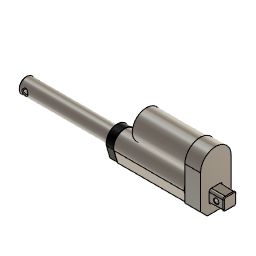
сборка v7 (Autodesk Fusion 360 archive; units mm, degrees)
design "actuators 10"
Autodesk Fusion 360 part; units mm, degrees
note: some values were not read from the file. Set by a fixed rule: which face or edge a step refers to.
sketch "Sketch1" plane through (0, 0, 0) normal (0, 0, 1) x (1, 0, 0)
  line L0 (8.5, 8.5) -> (-8.5, 8.5)
  line L1 (-8.5, 8.5) -> (-8.5, -8.5)
  line L2 (-8.5, -8.5) -> (8.5, -8.5)
  line L3 (8.5, -8.5) -> (8.5, 8.5)
  line L4 (8.5, 8.5) -> (-8.5, -8.5) construction
  line L5 (-8.5, 8.5) -> (8.5, -8.5) construction
  dimension "d1" = 17
  dimension "d2" = 17
  constraint horizontal L0
  constraint perpendicular L0 L1
  constraint parallel L0 L2
  constraint parallel L1 L3
  constraint coincident L4 origin
  constraint coincident L5 origin
  measures "d1" distance of L1.end L2.end
  measures "d2" distance of L0.end L1.end
ref_plane "WorkPlane1" through (0, 0, 19) normal (0, 0, 1) x (1, 0, 0)
sketch "Sketch2" plane through (0, 0, 19) normal (0, 0, 1) x (1, 0, 0)
  line L0 (9, 9) -> (-9, 9)
  line L1 (-9, 9) -> (-9, -9)
  line L2 (-9, -9) -> (9, -9)
  line L3 (9, -9) -> (9, 9)
  line L4 (9, 9) -> (-9, -9) construction
  line L5 (-9, 9) -> (9, -9) construction
  dimension "d4" = 18
  dimension "d5" = 18
  constraint horizontal L0
  constraint perpendicular L0 L1
  constraint parallel L0 L2
  constraint parallel L1 L3
  constraint coincident L4 origin
  constraint coincident L5 origin
  measures "d4" distance of L1.end L2.end
  measures "d5" distance of L0.end L1.end
loft "Loft1" add profiles "Sketch1", "Sketch2" section 1 section 2 makes body 1
fillet "Fillet1" radius 3 4 edges at (8.75, -8.75, 9.5) (-8.75, -8.75, 9.5) (-8.75, 8.75, 9.5) (8.75, 8.75, 9.5) on bodies 1
fillet "Fillet2" radius 1 1 faces at (-1.8337, -2.8333, 0) on bodies 1
sketch "Sketch3" plane through (0, 8.4941, -0.2235) normal (0, 0.999654, -0.026307) x (-1, 0, 0)
  line L0 (-5.5267, 1.1976) -> (5.5267, 1.1976)
  line L1 (5.5267, 1.1976) -> (6.001, 19.2302)
  line L2 (6.001, 19.2302) -> (-6.001, 19.2302)
  line L3 (-6.001, 19.2302) -> (-5.5267, 1.1976)
  line L4 (0, 0) -> (0, 6.5)
  line L5 (0, 6.5) -> (0.0789, 9.499)
  circle A0 centre (0.0789, 9.499) radius 3
  dimension "d10" = 6.5
  dimension "d11" = 3
  constraint coincident L4.start origin
  constraint perpendicular L0 L4
  constraint parallel L1 L5
  constraint coincident L5.end A0.centre
  constraint coincident L4.end A0
  measures "d10" distance of L4.start L4.end
  measures "d11" distance of L4.end L5.end
extrude "Extrude1" cut sketch "Sketch3" against normal blind 32 contours A0 bodies 1
fillet "Fillet3" radius 0.5 2 edges at (-0.0789, -8.8352, 12.7358) (2.7181, 8.7725, 10.3566) on bodies 1
sketch "Sketch4" plane through (0, 0, 19) normal (0, 0, 1) x (-1, 0, 0)
  ellipse E0 centre (-5.999, -5.999) end of major axis (-8.1218, -8.1218) minor radius 3 (-9, -6.001) -> (-6.001, -9) ccw
  line L0 (-6.001, -9) -> (6.001, -9)
  ellipse E1 centre (5.999, -5.999) end of major axis (8.1218, -8.1218) minor radius 3 (6.001, -9) -> (9, -6.001) ccw
  line L1 (9, -6.001) -> (9, 6.001)
  ellipse E2 centre (5.999, 5.999) end of major axis (8.1218, 8.1218) minor radius 3 (9, 6.001) -> (6.001, 9) ccw
  line L2 (6.001, 9) -> (-6.001, 9)
  ellipse E3 centre (-5.999, 5.999) end of major axis (-8.1218, 8.1218) minor radius 3 (-6.001, 9) -> (-9, 6.001) ccw
  line L3 (-9, 6.001) -> (-9, -6.001)
  line L4 (9, 0) -> (20.5, 0)
  line L5 (20.5, 0) -> (20.5, -11.5)
  line L6 (0, 0) -> (-39.2189, 0) construction
  line L7 (0, 0) -> (0, -20.5) construction
  line L8 (0, -20.5) -> (-34, -20.5)
  line L9 (20.5, -11.5) -> (11.5, -20.5)
  line L10 (20.5, -11.5) -> (33.2279, -11.5) construction
  line L11 (0, -20.5) -> (11.5, -20.5)
  line L12 (-54.5, 0) -> (-54.5, 0)
  arc A0 (-54.5, 0) -> (-34, -20.5) centre (-34, 0) ccw
  line L13 (20.5, 11.5) -> (11.5, 20.5)
  line L14 (20.5, 0) -> (20.5, 11.5)
  line L15 (0, 20.5) -> (11.5, 20.5)
  line L16 (0, 20.5) -> (-34, 20.5)
  arc A1 (-34, 20.5) -> (-54.5, 0) centre (-34, 0) ccw
  dimension "d16" = 11.5
  dimension "d17" = 11.5
  dimension "d19" = 20.5
  dimension "d23" = 135
  dimension "d25" = 20.5
  constraint midpoint L1 L4.start
  constraint perpendicular L1 L4
  constraint perpendicular L4 L5
  constraint coincident L6.start L7.start
  constraint horizontal L6
  constraint perpendicular L6 L7
  constraint perpendicular L7 L8
  constraint horizontal L10
  constraint tangent L8 A0
  constraint symmetric L4.end L6 L5.start
  constraint symmetric L5.end L6 L13.start
  constraint symmetric L6 L7.end L15.start
  constraint symmetric L6 L9.end L13.end
  constraint symmetric L6 L8.end L16.end
  constraint symmetric L6 L12.start L12.end
  constraint symmetric L6 A0 A1
  measures "d16" distance of L4.start L4.end
  measures "d17" distance of L4.end L5.end
  measures "d19" distance of L6.start L7.end
  measures "d23" angle of L9 L10
  measures "d25" radius of A0
extrude "Extrude2" add sketch "Sketch4" along normal blind 21 contours E0 L0 E1 L1 E2 L2 E3 L3 | L5 L8 L9 L11 A0 L13 L14 L15 L16 A1 bodies 1
sketch "Sketch5" plane through (0, 0, 40) normal (0, 0, 1) x (-1, 0, 0)
  line L0 (11.5, 20.5) -> (-34, 20.5)
  arc A0 (-34, 20.5) -> (-34, -20.5) centre (-34, 0) ccw
  line L1 (-34, -20.5) -> (11.5, -20.5)
  line L2 (11.5, -20.5) -> (20.5, -11.5)
  line L3 (20.5, -11.5) -> (20.5, 11.5)
  line L4 (20.5, 11.5) -> (11.5, 20.5)
  circle A1 centre (-34, 0) radius 19
  line L5 (0, 0) -> (20.5, 0) construction
  line L6 (20.5, 0) -> (20.5, -10)
  line L7 (20.5, -10) -> (20.5, -11.5)
  line L8 (0, 0) -> (1, 0)
  line L9 (0, 0) -> (0, 14.9666) construction
  line L10 (0, 0) -> (0, -14.9666) construction
  line L11 (0, 0) -> (15.2084, 0) construction
  line L12 (3.9362, -14.6901) -> (20.5, -10)
  arc A2 (-14, 0) -> (3.94, -14.7091) centre (1, 0) ccw
  line L13 (20.5, -11.5) -> (4.6077, -16)
  arc A3 (-13.5211, -7.6259) -> (4.6077, -16) centre (1, 0) ccw
  line L14 (1, 0) -> (-13.5211, -7.6259) construction
  line L15 (1, 0) -> (4.6077, -16) construction
  line L16 (-13.5211, -7.6259) -> (-12.2801, -6.9742)
  line L17 (3.9362, 14.6901) -> (20.5, 10)
  line L18 (20.5, 11.5) -> (4.6077, 16)
  arc A4 (3.94, 14.7091) -> (-14, 0) centre (1, 0) ccw
  arc A5 (4.6077, 16) -> (-13.5211, 7.6259) centre (1, 0) ccw
  line L19 (-13.5211, 7.6259) -> (-12.2801, 6.9742)
  line L20 (20.5, 0) -> (20.5, 10)
  line L21 (20.5, 10) -> (20.5, 11.5)
  arc A6 (-12.2801, -6.9742) -> (3.94, -14.7091) centre (1, 0) ccw
  arc A7 (3.94, 14.7091) -> (-12.2801, 6.9742) centre (1, 0) ccw
  line L22 (3.94, 14.7091) -> (4.3035, 16.0656)
  line L23 (3.94, 14.7091) -> (5.3444, 14.7091) construction
  line L24 (3.94, -14.7091) -> (4.3035, -16.0656)
  line L25 (20.5, -10) -> (20.5, -11.5)
  line L26 (20.5, 11.5) -> (20.5, 10)
  line L27 (20.5, 10) -> (3.94, 14.7091)
  line L28 (20.5, -10) -> (3.94, -14.7091)
  line L29 (20.5, -11.5) -> (4.3035, -16.0656)
  dimension "d28" = 38
  dimension "d29" = 10
  dimension "d30" = 1
  dimension "d33" = 15
  dimension "d34" = 75
  dimension "d35" = 75
  constraint concentric A0 A1
  constraint coincident L5.start L8.start
  constraint midpoint L3 L5.end
  constraint perpendicular L5 L6
  constraint coincident L2.end L3.start
  constraint parallel L5 L8
  constraint perpendicular L8 L9
  constraint perpendicular L8 L10
  constraint horizontal L11
  constraint coincident L8.end A2.centre
  constraint parallel L12 L13
  constraint coincident L14 L16.end
  constraint coincident A2 L16.end
  constraint symmetric L6.start L5 L20.start
  constraint symmetric L5 L6.end L17.end
  constraint symmetric L5 L2.end L3.end
  constraint symmetric L5 L12.start L17.start
  constraint symmetric L5 A2.start A4.end
  constraint symmetric L5 A2.end A4.start
  constraint symmetric L5 A2 A4
  constraint symmetric L5 L13.end L18.end
  constraint symmetric L5 A3.start A5.end
  constraint symmetric L5 A3 A5
  constraint symmetric L5 L16.end L19.end
  constraint horizontal L23
  constraint coincident A5 L22.end
  constraint symmetric L11 A4.start A2.end
  constraint symmetric L11 L22.end L24.end
  constraint coincident L3.end L4.start
  measures "d28" diameter of A1
  measures "d29" distance of L5.end L6.end
  measures "d30" distance of L5.start L8.end
  measures "d33" radius of A2
  measures "d34" angle of L14 L15
  measures "d35" angle of L22 L23
extrude "Extrude3" add sketch "Sketch5" along normal blind 5 contours L3 L18 A5 L21 L22 L26 L27 | A4 A5 L19 A7 L22 | L3 L7 L24 L25 L28 L29 | A2 A3 L16 A6 L24 bodies 1
extrude "Extrude4" add sketch "Sketch5" along normal blind 72 contours A1 bodies 1
extrude "Extrude5" add sketch "Sketch5" along normal blind 101 contours L3 L6 A2 A4 L20 A6 A7 L27 L28 bodies 1
extrude "Extrude6" add 1 faces at (-9.46, -3.3333, 141) along direction (0, 0, 1) blind 10 separate body on bodies 1 makes body 2
sketch "Sketch6" plane through (0, 0, 112) normal (0, 0, 1) x (-1, 0, 0)
  circle A0 centre (-34, 0) radius 19
  circle A1 centre (-34, 0) radius 6.25
  dimension "d44" = 12.5
  constraint concentric A0 A1
  measures "d44" diameter of A1
extrude "Extrude7" add sketch "Sketch6" along normal blind 3 contours A1 bodies 1
sketch "Sketch7" plane through (0, 0, 151) normal (0, 0, 1) x (-1, 0, 0)
  line L0 (20.5, -10) -> (20.5, 10)
  line L1 (20.5, 10) -> (3.94, 14.7091)
  arc A0 (3.94, 14.7091) -> (3.94, -14.7091) centre (1, 0) ccw
  line L2 (3.94, -14.7091) -> (20.5, -10)
  circle A1 centre (1, 0) radius 10
  dimension "d47" = 20
  constraint concentric A0 A1
  measures "d47" diameter of A1
extrude "Extrude8" add sketch "Sketch7" along normal blind 22.5 separate body contours A1 makes body 3
extrude "Extrude9" add 1 faces at (-4.1852, 0.9825, 151) along direction (0, 0, -1) blind 100 separate body on bodies 3 makes body 4
combine "Combine1" operation add target body 4 tool bodies 3
ref_plane "WorkPlane2" through (-1, -10, 164.9128) normal (0, -1, 0) x (1, 0, 0)
sketch "Sketch8" plane through (-1, -10, 164.9128) normal (0, -1, 0) x (1, 0, 0)
  line L0 (10, 8.5872) -> (-10, 8.5872)
  line L1 (-10, -113.9128) -> (10, -113.9128)
  line L2 (0, 8.5872) -> (0, 3.0872)
  line L3 (0, 3.0872) -> (0, 0.0872)
  circle A0 centre (0, 0.0872) radius 3
  dimension "d53" = 5.5
  dimension "d54" = 3
  constraint midpoint L0 L2.start
  constraint perpendicular L0 L2
  constraint parallel L2 L3
  constraint coincident L3.end A0.centre
  constraint coincident L2.end A0
  measures "d53" distance of L2.start L2.end
  measures "d54" distance of L2.end L3.end
extrude "Extrude10" cut sketch "Sketch8" against normal blind 33 bodies 4
fillet "Fillet4" radius 1 3 edges at (2, -9.5394, 165) (-4, -9.5394, 165) (-4, 9.5394, 165) on bodies 4
fillet "Fillet5" radius 1 1 edges at (8.3233, 3.6162, 173.5) on bodies 4
move_body "Move1" bodies 1 2 4 to x (0, 0, 1) y (0, 1, 0) z (-1, 0, 0) at (-20.508, 0, 20.492)
combine "Combine2" [no effect]
copy_body "Body->Comp1" bodies 1 removing the originals makes body 5 in component "Component"
copy_body "Body->Comp5" bodies 4 removing the originals makes body 6 in component "Component'"
copy_body "Body->Comp6" bodies 2 removing the originals makes body 7 in component "Component''"
move_body "Move1'" bodies 6 to x (1, 0, 0) y (0, 1, 0) z (0, 0, 1) at (-100, 0, 0) in component "Component'"
component "Component" placed x (1, 0, 0) y (0, 1, 0) z (0, 0, 1) at (0, 0, 0)
component "Component'" placed x (1, 0, 0) y (0, 1, 0) z (0, 0, 1) at (0, 0, -0.728)
component "Component''" placed x (1, 0, 0) y (0, 1, 0) z (0, 0, 1) at (0, 0, 0)

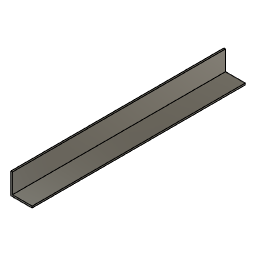
design "Уголок_3"
Autodesk Fusion 360 part; units mm, degrees
sketch "Sketch1" plane through (0, 0, 0) normal (0, 1, 0) x (1, 0, 0)
  line L0 (0, 0) -> (0, -40)
  line L1 (0, 0) -> (40, 0)
  line L2 (40, 0) -> (40, -3)
  line L3 (0, -40) -> (3, -40)
  line L4 (3, -40) -> (3, -3)
  line L5 (3, -3) -> (40, -3)
  dimension "d1" = 40
  dimension "d2" = 40
  dimension "d3" = 3
  dimension "d4" = 3
  constraint coincident L0.start L1.start
  constraint vertical L0
  constraint perpendicular L0 L1
  constraint perpendicular L1 L2
  constraint perpendicular L0 L3
  constraint perpendicular L1 L4
  constraint perpendicular L2 L5
  measures "d1" distance of L0.start L0.end
  measures "d2" distance of L0.start L1.end
  measures "d3" distance of L1.end L2.end
  measures "d4" distance of L0.end L3.end
extrude "Extrude1" add sketch "Sketch1" against normal blind 425
extrude "Extrude2" add 1 faces at (1, -425, 14.3333) along direction (0, -1, 0) blind 375
extrude "Extrude3" cut 1 faces at (1, -800, 14.3333) along direction (0, 1, 0) blind 50
extrude "Extrude4" cut 1 faces at (1, 0, 14.3333) along direction (0, -1, 0) blind 350

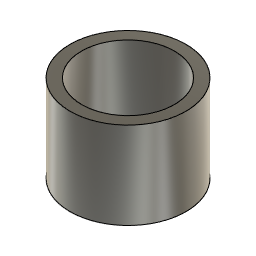
design "подставки под нагреватель"
Autodesk Fusion 360 part; units mm, degrees
sketch "Sketch1" plane through (0, 0, 0) normal (0, 0, 1) x (1, 0, 0)
  circle A0 centre (0, 0) radius 10
  circle A1 centre (0, 0) radius 8
  dimension "d1" = 20
  dimension "d2" = 16
  constraint coincident A0.centre A1.centre
  constraint concentric A0 A1
  measures "d1" diameter of A0
  measures "d2" diameter of A1
extrude "Extrude1" add sketch "Sketch1" along normal blind 15

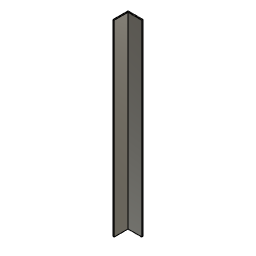
design "Уголок_вертикальный"
Autodesk Fusion 360 part; units mm, degrees
sketch "Sketch1" plane through (0, 0, 0) normal (0, 1, 0) x (1, 0, 0)
  line L0 (0, 0) -> (0, -40)
  line L1 (0, 0) -> (40, 0)
  line L2 (40, 0) -> (40, -3)
  line L3 (0, -40) -> (3, -40)
  line L4 (3, -40) -> (3, -3)
  line L5 (3, -3) -> (40, -3)
  dimension "d1" = 40
  dimension "d2" = 40
  dimension "d3" = 3
  dimension "d4" = 3
  constraint coincident L0.start L1.start
  constraint vertical L0
  constraint perpendicular L0 L1
  constraint perpendicular L1 L2
  constraint perpendicular L0 L3
  constraint perpendicular L1 L4
  constraint perpendicular L2 L5
  measures "d1" distance of L0.start L0.end
  measures "d2" distance of L0.start L1.end
  measures "d3" distance of L1.end L2.end
  measures "d4" distance of L0.end L3.end
extrude "Extrude1" add sketch "Sketch1" against normal blind 500
move_body "Move1" bodies 1 to x (1, 0, 0) y (0, 0, 1) z (0, -1, 0) at (0, -800, 800)

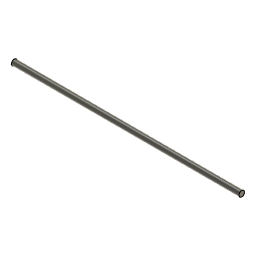
design "оси"
Autodesk Fusion 360 part; units mm, degrees
sketch "Sketch1" plane through (0, 0, 0) normal (1, 0, 0) x (0, 1, 0)
  circle A0 centre (0, 0) radius 3
  dimension "d1" = 6
  constraint coincident A0.centre origin
  measures "d1" diameter of A0
extrude "Extrude1" add sketch "Sketch1" along normal blind 243

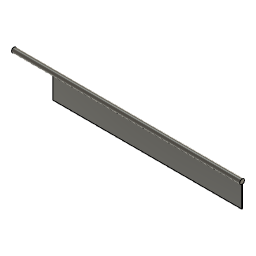
design "ось лопатка"
Autodesk Fusion 360 part; units mm, degrees
sketch "Sketch1" plane through (0, 0, 0) normal (1, 0, 0) x (0, 1, 0)
  circle A0 centre (0, 0) radius 3
  line L0 (0, 0) -> (0, -50) construction
  line L1 (0, 0) -> (0.5, 0)
  line L2 (0, -50) -> (-0.5, -50)
  line L3 (-0.5, -50) -> (0.5, -50)
  line L4 (0.5, -50) -> (0.5, 0)
  line L5 (0.5, 0) -> (-0.5, 0)
  line L6 (-0.5, 0) -> (-0.5, -50)
  dimension "d1" = 6
  dimension "d4" = 50
  dimension "d5" = 0.5
  dimension "d6" = 0.5
  constraint coincident A0.centre L0.start
  constraint vertical L0
  constraint perpendicular L0 L1
  constraint perpendicular L0 L2
  constraint horizontal L3
  constraint vertical L4
  constraint horizontal L5
  constraint vertical L6
  measures "d1" diameter of A0
  measures "d4" distance of A0.centre L0.end
  measures "d5" distance of A0.centre L1.end
  measures "d6" distance of L0.end L2.end
extrude "Extrude1" add sketch "Sketch1" along normal blind 360
sketch "Sketch2" plane through (360, 0, 0) normal (1, 0, 0) x (0, 1, 0)
  arc A0 (0.5, -2.958) -> (-0.5, -2.958) centre (0, 0) ccw
  line L0 (-0.5, -2.958) -> (-0.5, -50)
  line L1 (-0.5, -50) -> (0.5, -50)
  line L2 (0.5, -50) -> (0.5, -2.958)
  line L3 (-0.5, -2.958) -> (0.5, -2.958)
  line L4 (0.5, -2.958) -> (0.5, -50)
  line L5 (0.5, -50) -> (-0.5, -50)
  line L6 (-0.5, -50) -> (-0.5, -2.958)
  constraint horizontal L3
  constraint vertical L4
  constraint horizontal L5
  constraint vertical L6
  constraint coincident L1.end L2.start
  constraint coincident A0.end L0.start
extrude "Extrude2" cut sketch "Sketch2" against normal blind 50 contours L0 L1 L2 L3 L4 L5 L6
sketch "Sketch3" plane through (0, 0, 0) normal (-1, 0, 0) x (0, -1, 0)
  arc A0 (0.5, -2.958) -> (-0.5, -2.958) centre (0, 0) ccw
  line L0 (-0.5, -2.958) -> (-0.5, -50)
  line L1 (-0.5, -50) -> (0.5, -50)
  line L2 (0.5, -50) -> (0.5, -2.958)
  line L3 (-0.5, -2.958) -> (0.5, -2.958)
  line L4 (0.5, -2.958) -> (0.5, -50)
  line L5 (0.5, -50) -> (-0.5, -50)
  line L6 (-0.5, -50) -> (-0.5, -2.958)
  constraint horizontal L3
  constraint vertical L4
  constraint horizontal L5
  constraint vertical L6
  constraint coincident L1.end L2.start
  constraint coincident A0.end L0.start
extrude "Extrude3" cut sketch "Sketch3" against normal blind 50 contours L0 L1 L2 L3 L4 L5 L6
extrude "Extrude4" cut 2 faces at (223.3333, 0.1667, -50) (223.3333, -0.1667, -50) along direction (0, 0, 1) blind 20
extrude "Extrude5" cut 1 faces at (50, 0, -11.972) along direction (1, 0, 0) blind 20
extrude "Extrude6" cut 1 faces at (0, 0.7466, 0.5854) along direction (1, 0, 0) blind 20
extrude "Extrude7" cut 1 faces at (360, 0.7466, 0.5854) along direction (-1, 0, 0) blind 50

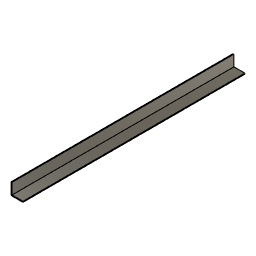
design "Уголок"
Autodesk Fusion 360 part; units mm, degrees
sketch "Sketch1" plane through (0, 0, 0) normal (0, 1, 0) x (1, 0, 0)
  line L0 (0, 0) -> (0, -40)
  line L1 (0, 0) -> (40, 0)
  line L2 (40, 0) -> (40, -3)
  line L3 (0, -40) -> (3, -40)
  line L4 (3, -40) -> (3, -3)
  line L5 (3, -3) -> (40, -3)
  dimension "d1" = 40
  dimension "d2" = 40
  dimension "d3" = 3
  dimension "d4" = 3
  constraint coincident L0.start L1.start
  constraint vertical L0
  constraint perpendicular L0 L1
  constraint perpendicular L1 L2
  constraint perpendicular L0 L3
  constraint perpendicular L1 L4
  constraint perpendicular L2 L5
  measures "d1" distance of L0.start L0.end
  measures "d2" distance of L0.start L1.end
  measures "d3" distance of L1.end L2.end
  measures "d4" distance of L0.end L3.end
extrude "Extrude1" add sketch "Sketch1" against normal blind 425
extrude "Extrude2" add 1 faces at (1, -425, 14.3333) along direction (0, -1, 0) blind 375
extrude "Extrude3" cut 1 faces at (1, -800, 14.3333) along direction (0, 1, 0) blind 50

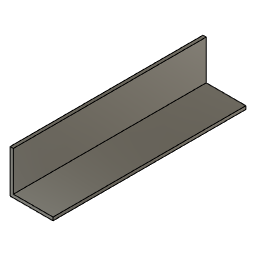
design "уголок_3"
Autodesk Fusion 360 part; units mm, degrees
sketch "Sketch1" plane through (0, 0, 0) normal (0, 1, 0) x (1, 0, 0)
  line L0 (0, 0) -> (0, -40)
  line L1 (0, 0) -> (40, 0)
  line L2 (40, 0) -> (40, -3)
  line L3 (0, -40) -> (3, -40)
  line L4 (3, -40) -> (3, -3)
  line L5 (3, -3) -> (40, -3)
  dimension "d1" = 40
  dimension "d2" = 40
  dimension "d3" = 3
  dimension "d4" = 3
  constraint coincident L0.start L1.start
  constraint vertical L0
  constraint perpendicular L0 L1
  constraint perpendicular L1 L2
  constraint perpendicular L0 L3
  constraint perpendicular L1 L4
  constraint perpendicular L2 L5
  measures "d1" distance of L0.start L0.end
  measures "d2" distance of L0.start L1.end
  measures "d3" distance of L1.end L2.end
  measures "d4" distance of L0.end L3.end
extrude "Extrude1" add sketch "Sketch1" along normal blind 200
extrude "Extrude4" cut 1 faces at (1, 0, 14.3333) along direction (0, 1, 0) blind 20

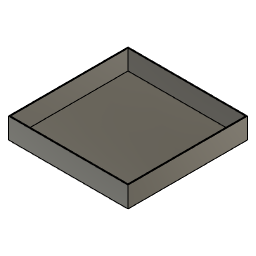
design "ванна"
Autodesk Fusion 360 part; units mm, degrees
sketch "Sketch1" plane through (0, 0, 0) normal (0, 0, 1) x (1, 0, 0)
  line L0 (122.5, 122.5) -> (-122.5, 122.5)
  line L1 (-122.5, 122.5) -> (-122.5, -122.5)
  line L2 (-122.5, -122.5) -> (122.5, -122.5)
  line L3 (122.5, -122.5) -> (122.5, 122.5)
  line L4 (122.5, 122.5) -> (-122.5, -122.5) construction
  line L5 (-122.5, 122.5) -> (122.5, -122.5) construction
  line L6 (120.5, 120.5) -> (-120.5, 120.5)
  line L7 (-120.5, 120.5) -> (-120.5, -120.5)
  line L8 (-120.5, -120.5) -> (120.5, -120.5)
  line L9 (120.5, -120.5) -> (120.5, 120.5)
  line L10 (120.5, 120.5) -> (-120.5, -120.5) construction
  line L11 (-120.5, 120.5) -> (120.5, -120.5) construction
  dimension "d1" = 245
  dimension "d2" = 245
  dimension "d3" = 241
  dimension "d4" = 241
  constraint horizontal L0
  constraint perpendicular L0 L1
  constraint parallel L0 L2
  constraint parallel L1 L3
  constraint coincident L4 origin
  constraint coincident L5 origin
  constraint horizontal L6
  constraint perpendicular L6 L7
  constraint parallel L6 L8
  constraint parallel L7 L9
  constraint coincident L10 origin
  constraint coincident L11 origin
  measures "d1" distance of L0.end L1.end
  measures "d2" distance of L1.end L2.end
  measures "d3" distance of L7.end L8.end
  measures "d4" distance of L6.end L7.end
extrude "Extrude1" add sketch "Sketch1" along normal blind 42.5
extrude "Extrude2" add sketch "Sketch1" along normal blind 2 contours L6 L7 L8 L9

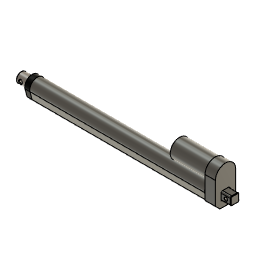
design "actuators 30"
Autodesk Fusion 360 part; units mm, degrees
sketch "Sketch1" plane through (0, 0, 0) normal (0, 0, 1) x (1, 0, 0)
  line L0 (8.5, 8.5) -> (-8.5, 8.5)
  line L1 (-8.5, 8.5) -> (-8.5, -8.5)
  line L2 (-8.5, -8.5) -> (8.5, -8.5)
  line L3 (8.5, -8.5) -> (8.5, 8.5)
  line L4 (8.5, 8.5) -> (-8.5, -8.5) construction
  line L5 (-8.5, 8.5) -> (8.5, -8.5) construction
  dimension "d1" = 17
  dimension "d2" = 17
  constraint horizontal L0
  constraint perpendicular L0 L1
  constraint parallel L0 L2
  constraint parallel L1 L3
  constraint coincident L4 origin
  constraint coincident L5 origin
  measures "d1" distance of L1.end L2.end
  measures "d2" distance of L0.end L1.end
ref_plane "WorkPlane1" through (0, 0, 19) normal (0, 0, 1) x (1, 0, 0)
sketch "Sketch2" plane through (0, 0, 19) normal (0, 0, 1) x (1, 0, 0)
  line L0 (9, 9) -> (-9, 9)
  line L1 (-9, 9) -> (-9, -9)
  line L2 (-9, -9) -> (9, -9)
  line L3 (9, -9) -> (9, 9)
  line L4 (9, 9) -> (-9, -9) construction
  line L5 (-9, 9) -> (9, -9) construction
  dimension "d4" = 18
  dimension "d5" = 18
  constraint horizontal L0
  constraint perpendicular L0 L1
  constraint parallel L0 L2
  constraint parallel L1 L3
  constraint coincident L4 origin
  constraint coincident L5 origin
  measures "d4" distance of L1.end L2.end
  measures "d5" distance of L0.end L1.end
loft "Loft1" add profiles "Sketch1", "Sketch2" section 1 section 2 makes body 1
fillet "Fillet1" radius 3 4 edges at (8.75, -8.75, 9.5) (-8.75, -8.75, 9.5) (-8.75, 8.75, 9.5) (8.75, 8.75, 9.5) on bodies 1
fillet "Fillet2" radius 1 1 faces at (-1.8337, -2.8333, 0) on bodies 1
sketch "Sketch3" plane through (0, 8.4941, -0.2235) normal (0, 0.999654, -0.026307) x (-1, 0, 0)
  line L0 (-5.5267, 1.1976) -> (5.5267, 1.1976)
  line L1 (5.5267, 1.1976) -> (6.001, 19.2302)
  line L2 (6.001, 19.2302) -> (-6.001, 19.2302)
  line L3 (-6.001, 19.2302) -> (-5.5267, 1.1976)
  line L4 (0, 0) -> (0, 6.5)
  line L5 (0, 6.5) -> (0.0789, 9.499)
  circle A0 centre (0.0789, 9.499) radius 3
  dimension "d10" = 6.5
  dimension "d11" = 3
  constraint coincident L4.start origin
  constraint perpendicular L0 L4
  constraint parallel L1 L5
  constraint coincident L5.end A0.centre
  constraint coincident L4.end A0
  measures "d10" distance of L4.start L4.end
  measures "d11" distance of L4.end L5.end
extrude "Extrude1" cut sketch "Sketch3" against normal blind 32 contours A0 bodies 1
fillet "Fillet3" radius 0.5 2 edges at (-0.0789, -8.8352, 12.7358) (2.7181, 8.7725, 10.3566) on bodies 1
sketch "Sketch4" plane through (0, 0, 19) normal (0, 0, 1) x (-1, 0, 0)
  ellipse E0 centre (-5.999, -5.999) end of major axis (-8.1218, -8.1218) minor radius 3 (-9, -6.001) -> (-6.001, -9) ccw
  line L0 (-6.001, -9) -> (6.001, -9)
  ellipse E1 centre (5.999, -5.999) end of major axis (8.1218, -8.1218) minor radius 3 (6.001, -9) -> (9, -6.001) ccw
  line L1 (9, -6.001) -> (9, 6.001)
  ellipse E2 centre (5.999, 5.999) end of major axis (8.1218, 8.1218) minor radius 3 (9, 6.001) -> (6.001, 9) ccw
  line L2 (6.001, 9) -> (-6.001, 9)
  ellipse E3 centre (-5.999, 5.999) end of major axis (-8.1218, 8.1218) minor radius 3 (-6.001, 9) -> (-9, 6.001) ccw
  line L3 (-9, 6.001) -> (-9, -6.001)
  line L4 (9, 0) -> (20.5, 0)
  line L5 (20.5, 0) -> (20.5, -11.5)
  line L6 (0, 0) -> (-39.2189, 0) construction
  line L7 (0, 0) -> (0, -20.5) construction
  line L8 (0, -20.5) -> (-34, -20.5)
  line L9 (20.5, -11.5) -> (11.5, -20.5)
  line L10 (20.5, -11.5) -> (33.2279, -11.5) construction
  line L11 (0, -20.5) -> (11.5, -20.5)
  line L12 (-54.5, 0) -> (-54.5, 0)
  arc A0 (-54.5, 0) -> (-34, -20.5) centre (-34, 0) ccw
  line L13 (20.5, 11.5) -> (11.5, 20.5)
  line L14 (20.5, 0) -> (20.5, 11.5)
  line L15 (0, 20.5) -> (11.5, 20.5)
  line L16 (0, 20.5) -> (-34, 20.5)
  arc A1 (-34, 20.5) -> (-54.5, 0) centre (-34, 0) ccw
  dimension "d16" = 11.5
  dimension "d17" = 11.5
  dimension "d19" = 20.5
  dimension "d23" = 135
  dimension "d25" = 20.5
  constraint midpoint L1 L4.start
  constraint perpendicular L1 L4
  constraint perpendicular L4 L5
  constraint coincident L6.start L7.start
  constraint horizontal L6
  constraint perpendicular L6 L7
  constraint perpendicular L7 L8
  constraint horizontal L10
  constraint tangent L8 A0
  constraint symmetric L4.end L6 L5.start
  constraint symmetric L5.end L6 L13.start
  constraint symmetric L6 L7.end L15.start
  constraint symmetric L6 L9.end L13.end
  constraint symmetric L6 L8.end L16.end
  constraint symmetric L6 L12.start L12.end
  constraint symmetric L6 A0 A1
  measures "d16" distance of L4.start L4.end
  measures "d17" distance of L4.end L5.end
  measures "d19" distance of L6.start L7.end
  measures "d23" angle of L9 L10
  measures "d25" radius of A0
extrude "Extrude2" add sketch "Sketch4" along normal blind 21 contours E0 L0 E1 L1 E2 L2 E3 L3 | L5 L8 L9 L11 A0 L13 L14 L15 L16 A1 bodies 1
sketch "Sketch5" plane through (0, 0, 40) normal (0, 0, 1) x (-1, 0, 0)
  line L0 (11.5, 20.5) -> (-34, 20.5)
  arc A0 (-34, 20.5) -> (-34, -20.5) centre (-34, 0) ccw
  line L1 (-34, -20.5) -> (11.5, -20.5)
  line L2 (11.5, -20.5) -> (20.5, -11.5)
  line L3 (20.5, -11.5) -> (20.5, 11.5)
  line L4 (20.5, 11.5) -> (11.5, 20.5)
  circle A1 centre (-34, 0) radius 19
  line L5 (0, 0) -> (20.5, 0) construction
  line L6 (20.5, 0) -> (20.5, -10)
  line L7 (20.5, -10) -> (20.5, -11.5)
  line L8 (0, 0) -> (1, 0)
  line L9 (0, 0) -> (0, 14.9666) construction
  line L10 (0, 0) -> (0, -14.9666) construction
  line L11 (0, 0) -> (15.2084, 0) construction
  line L12 (3.9362, -14.6901) -> (20.5, -10)
  arc A2 (-14, 0) -> (3.94, -14.7091) centre (1, 0) ccw
  line L13 (20.5, -11.5) -> (4.6077, -16)
  arc A3 (-13.5211, -7.6259) -> (4.6077, -16) centre (1, 0) ccw
  line L14 (1, 0) -> (-13.5211, -7.6259) construction
  line L15 (1, 0) -> (4.6077, -16) construction
  line L16 (-13.5211, -7.6259) -> (-12.2801, -6.9742)
  line L17 (3.9362, 14.6901) -> (20.5, 10)
  line L18 (20.5, 11.5) -> (4.6077, 16)
  arc A4 (3.94, 14.7091) -> (-14, 0) centre (1, 0) ccw
  arc A5 (4.6077, 16) -> (-13.5211, 7.6259) centre (1, 0) ccw
  line L19 (-13.5211, 7.6259) -> (-12.2801, 6.9742)
  line L20 (20.5, 0) -> (20.5, 10)
  line L21 (20.5, 10) -> (20.5, 11.5)
  arc A6 (-12.2801, -6.9742) -> (3.94, -14.7091) centre (1, 0) ccw
  arc A7 (3.94, 14.7091) -> (-12.2801, 6.9742) centre (1, 0) ccw
  line L22 (3.94, 14.7091) -> (4.3035, 16.0656)
  line L23 (3.94, 14.7091) -> (5.3444, 14.7091) construction
  line L24 (3.94, -14.7091) -> (4.3035, -16.0656)
  line L25 (20.5, -10) -> (20.5, -11.5)
  line L26 (20.5, 11.5) -> (20.5, 10)
  line L27 (20.5, 10) -> (3.94, 14.7091)
  line L28 (20.5, -10) -> (3.94, -14.7091)
  line L29 (20.5, -11.5) -> (4.3035, -16.0656)
  dimension "d28" = 38
  dimension "d29" = 10
  dimension "d30" = 1
  dimension "d33" = 15
  dimension "d34" = 75
  dimension "d35" = 75
  constraint concentric A0 A1
  constraint coincident L5.start L8.start
  constraint midpoint L3 L5.end
  constraint perpendicular L5 L6
  constraint coincident L2.end L3.start
  constraint parallel L5 L8
  constraint perpendicular L8 L9
  constraint perpendicular L8 L10
  constraint horizontal L11
  constraint coincident L8.end A2.centre
  constraint parallel L12 L13
  constraint coincident L14 L16.end
  constraint coincident A2 L16.end
  constraint symmetric L6.start L5 L20.start
  constraint symmetric L5 L6.end L17.end
  constraint symmetric L5 L2.end L3.end
  constraint symmetric L5 L12.start L17.start
  constraint symmetric L5 A2.start A4.end
  constraint symmetric L5 A2.end A4.start
  constraint symmetric L5 A2 A4
  constraint symmetric L5 L13.end L18.end
  constraint symmetric L5 A3.start A5.end
  constraint symmetric L5 A3 A5
  constraint symmetric L5 L16.end L19.end
  constraint horizontal L23
  constraint coincident A5 L22.end
  constraint symmetric L11 A4.start A2.end
  constraint symmetric L11 L22.end L24.end
  constraint coincident L3.end L4.start
  measures "d28" diameter of A1
  measures "d29" distance of L5.end L6.end
  measures "d30" distance of L5.start L8.end
  measures "d33" radius of A2
  measures "d34" angle of L14 L15
  measures "d35" angle of L22 L23
extrude "Extrude3" add sketch "Sketch5" along normal blind 5 contours L3 L18 A5 L21 L22 L26 L27 | A4 A5 L19 A7 L22 | L3 L7 L24 L25 L28 L29 | A2 A3 L16 A6 L24 bodies 1
extrude "Extrude4" add sketch "Sketch5" along normal blind 72 contours A1 bodies 1
extrude "Extrude5" add sketch "Sketch5" along normal blind 101 contours L3 L6 A2 A4 L20 A6 A7 L27 L28 bodies 1
extrude "Extrude6" add 1 faces at (-9.46, -3.3333, 141) along direction (0, 0, 1) blind 10 separate body on bodies 1 makes body 2
sketch "Sketch6" plane through (0, 0, 112) normal (0, 0, 1) x (-1, 0, 0)
  circle A0 centre (-34, 0) radius 19
  circle A1 centre (-34, 0) radius 6.25
  dimension "d44" = 12.5
  constraint concentric A0 A1
  measures "d44" diameter of A1
extrude "Extrude7" add sketch "Sketch6" along normal blind 3 contours A1 bodies 1
sketch "Sketch7" plane through (0, 0, 151) normal (0, 0, 1) x (-1, 0, 0)
  line L0 (20.5, -10) -> (20.5, 10)
  line L1 (20.5, 10) -> (3.94, 14.7091)
  arc A0 (3.94, 14.7091) -> (3.94, -14.7091) centre (1, 0) ccw
  line L2 (3.94, -14.7091) -> (20.5, -10)
  circle A1 centre (1, 0) radius 10
  dimension "d47" = 20
  constraint concentric A0 A1
  measures "d47" diameter of A1
extrude "Extrude8" add sketch "Sketch7" along normal blind 22.5 separate body contours A1 makes body 3
extrude "Extrude9" add 1 faces at (-4.1852, 0.9825, 151) along direction (0, 0, -1) blind 100 separate body on bodies 3 makes body 4
combine "Combine1" operation add target body 4 tool bodies 3
ref_plane "WorkPlane2" through (-1, -10, 164.9128) normal (0, -1, 0) x (1, 0, 0)
sketch "Sketch8" plane through (-1, -10, 164.9128) normal (0, -1, 0) x (1, 0, 0)
  line L0 (10, 8.5872) -> (-10, 8.5872)
  line L1 (-10, -113.9128) -> (10, -113.9128)
  line L2 (0, 8.5872) -> (0, 3.0872)
  line L3 (0, 3.0872) -> (0, 0.0872)
  circle A0 centre (0, 0.0872) radius 3
  dimension "d53" = 5.5
  dimension "d54" = 3
  constraint midpoint L0 L2.start
  constraint perpendicular L0 L2
  constraint parallel L2 L3
  constraint coincident L3.end A0.centre
  constraint coincident L2.end A0
  measures "d53" distance of L2.start L2.end
  measures "d54" distance of L2.end L3.end
extrude "Extrude10" cut sketch "Sketch8" against normal blind 33 bodies 4
fillet "Fillet4" radius 1 3 edges at (2, -9.5394, 165) (-4, -9.5394, 165) (-4, 9.5394, 165) on bodies 4
fillet "Fillet5" radius 1 1 edges at (8.3233, 3.6162, 173.5) on bodies 4
move_body "Move1" bodies 1 2 4 to x (0, 0, 1) y (0, 1, 0) z (-1, 0, 0) at (-20.508, 0, 20.492)
copy_body "CopyPasteBodies1" bodies 1 2 4 makes body 5 makes body 6 makes body 7
move_body "Move2" bodies 5 6 7 to x (1, 0, 0) y (0, 1, 0) z (0, 0, 1) at (0, 120, 0)
move_body "Move3" bodies 7 to x (1, 0, 0) y (0, 1, 0) z (0, 0, 1) at (-300, 0, 0)
move_body "Move4" bodies 6 to x (1, 0, 0) y (0, 1, 0) z (0, 0, 1) at (-200, 0, 0)
extrude "Extrude11" add 1 faces at (-161.508, 123.3333, 11.032) along direction (-1, 0, 0) blind 259 separate body on bodies 5 makes body 8
move_body "Move5" bodies 6 to x (1, 0, 0) y (0, 1, 0) z (0, 0, 1) at (-66, 0, 0)
move_body "Move6" bodies 6 to x (1, 0, 0) y (0, 1, 0) z (0, 0, 1) at (7, 0, 0)
move_body "Move7" bodies 7 to x (1, 0, 0) y (0, 1, 0) z (0, 0, 1) at (-475, 0, 0)
extrude "Extrude12" add 1 faces at (-846.508, 120.4638, 20.1722) along direction (1, 0, 0) blind 200 on bodies 7 bodies 7
combine "Combine2" operation add target body 8 tool bodies 5
move_body "Move8" bodies 7 to x (1, 0, 0) y (0, 1, 0) z (0, 0, 1) at (500, 0, 0)
copy_body "Body->Comp2" bodies 8 removing the originals makes body 9 in component "Component"
copy_body "Body->Comp3" bodies 6 removing the originals makes body 10 in component "Component'"
copy_body "Body->Comp4" bodies 7 removing the originals makes body 11 in component "Component''"
move_body "Move1'" bodies 11 to x (1, 0, 0) y (0, 1, 0) z (0, 0, 1) at (-285, 0, 0) in component "Component''"
component "Component" placed x (1, 0, 0) y (0, 1, 0) z (0, 0, 1) at (0, 0, 0)
component "Component'" placed x (1, 0, 0) y (0, 1, 0) z (0, 0, 1) at (0, 0, 0)
component "Component''" placed x (1, 0, 0) y (0, 1, 0) z (0, 0, 1) at (301, 0, -0.728)
hidden bodies 2 4 1

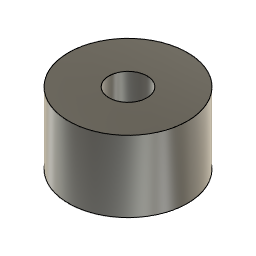
design "ножка"
Autodesk Fusion 360 part; units mm, degrees
sketch "Sketch1" plane through (0, 0, 0) normal (0, 0, 1) x (1, 0, 0)
  circle A0 centre (0, 0) radius 12.5
  circle A1 centre (0, 0) radius 4
  dimension "d1" = 25
  dimension "d2" = 8
  constraint coincident A0.centre A1.centre
  measures "d1" diameter of A0
  measures "d2" diameter of A1
extrude "Extrude1" add sketch "Sketch1" along normal blind 15

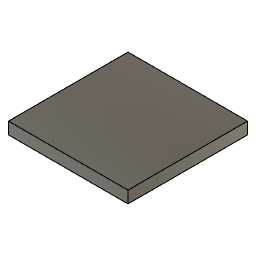
design "нагреватель"
Autodesk Fusion 360 part; units mm, degrees
sketch "Sketch1" plane through (0, 0, 0) normal (0, 0, 1) x (1, 0, 0)
  line L0 (150, 150) -> (-150, 150)
  line L1 (-150, 150) -> (-150, -150)
  line L2 (-150, -150) -> (150, -150)
  line L3 (150, -150) -> (150, 150)
  line L4 (150, 150) -> (-150, -150) construction
  line L5 (-150, 150) -> (150, -150) construction
  dimension "d1" = 300
  dimension "d2" = 300
  constraint horizontal L0
  constraint perpendicular L0 L1
  constraint parallel L0 L2
  constraint parallel L1 L3
  constraint coincident L4 origin
  constraint coincident L5 origin
  measures "d1" distance of L1.end L2.end
  measures "d2" distance of L0.end L1.end
extrude "Extrude1" add sketch "Sketch1" along normal blind 30
